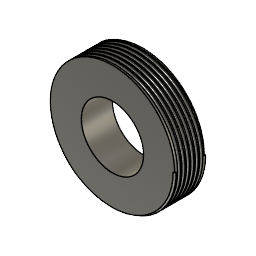
OutputDrum (Autodesk Fusion 360 design; units mm, degrees)
part number: 2026-02-01-13-44-55-001
Autodesk Fusion 360 part; units mm, degrees
sketch "Sketch1" plane through (0, 0, 0) normal (0, 1, 0) x (1, 0, 0)
  circle A0 centre (0, 0) radius 80
  dimension "d3" = 160
  constraint coincident A0.centre origin
  measures "d3" diameter of A0
extrude "Extrude1" add sketch "Sketch1" along normal mid plane 40
sketch "Sketch2" plane through (0, -20, 0) normal (0, -1, 0) x (1, 0, 0)
  circle A0 centre (0, 0) radius 40
  circle A1 centre (0, 0) radius 80
  dimension "d7" = 80
  constraint coincident A0.centre A1.centre
  measures "d7" diameter of A0
extrude "Extrude2" cut sketch "Sketch2" against normal through all contours A0
coil "CoilPrimitive1" cut diameter 160 section circle size 4 on centre turns 7 pitch 5.71429 right hand placed x (1, 0, 0) y (0, 0, -1) z (0, 1, 0) at (0, -20, 0)
equation "outputR = 80 mm"
equation "outputL = 40 mm"
equation "d3 = 2 * outputR"
equation "d4 = outputL"
equation "OD = 80 mm"
equation "d7 = OD"
equation "d10 = 2 * outputR"
equation "d14 = -outputL"
